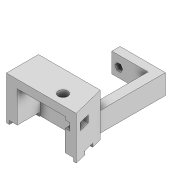
# Autodesk Inventor part: Part2
Saved by Autodesk Inventor 2022 (Build 260153000, 153)
## iProperties
Created: 2021-06-22
Part Number: Part2
Material: Generic
Document SubType Name: Modeling
Designer: Prajwal Patil
Density: 1 g/cm^3
Appearance: Default
Author: Prajwal Patil
Autodesk Inventor part; units mm, degrees
ref_plane "YZ Plane" through (0, 0, 0) normal (1, 0, 0) x (0, 1, 0)
ref_plane "XZ Plane" through (0, 0, 0) normal (0, 1, 0) x (-1, 0, 0)
sketch "Sketch1" plane through (0, 0, 0) normal (0, 0, 1) x (1, 0, 0)
  line L0 (-33.8514, 24.552) -> (33.4586, 24.552)
  line L1 (33.4586, 24.552) -> (33.4586, -22.438)
  line L2 (33.4586, -22.438) -> (-33.8514, -22.438)
  line L3 (-33.8514, -22.438) -> (-33.8514, 24.552)
  line L4 (33.4586, -22.438) -> (33.4586, -16.088)
  line L5 (33.4586, -16.088) -> (23.2986, -16.088)
  line L6 (23.2986, -16.088) -> (23.2986, 5.502)
  line L7 (23.2986, 5.502) -> (33.4586, 5.502)
  point P0 (0, 0)
  dimension "d0" = 67.31
  dimension "d1" = 46.99
  dimension "d10" = 6.35
  dimension "d11" = 10.16
  dimension "d12" = 21.59
  constraints: 16 end point, 4 perpendicular, 2 parallel, 2 point on line, 1 horizontal
  measures "d0" distance of L1.end L2.end
  measures "d1" distance of L0.end L1.end
  measures "d10" distance of L1.end L4.end
  measures "d11" distance of L4.end L5.end
  measures "d12" distance of L5.end L6.end
ref_plane "Work Plane3" through (-33.8514, -22.438, 0) normal (0, 0, 1) x (0, 1, 0)
ref_plane "Work Plane4" through (-33.8514, -22.438, 35.052) normal (0, 0, 1) x (0, 1, 0)
sketch "Sketch3" plane through (-33.8514, -22.438, 35.052) normal (0, 0, 1) x (0, 1, 0)
  line L0 (0, 0) -> (46.99, 0)
  line L1 (46.99, 0) -> (46.99, -76.2)
  line L2 (46.99, -76.2) -> (0, -76.2)
  line L3 (0, -76.2) -> (0, 0)
  point P0 (22.438, -33.8514)
  dimension "d4" = 46.99
  dimension "d5" = 76.2
  constraints: 8 end point, 2 parallel, 1 horizontal, 1 perpendicular
  measures "d4" distance of L1.end L2.end
  measures "d5" distance of L0.end L1.end
loft "Loft1" add profiles "Sketch3", "Sketch1"
sketch "Sketch5" plane through (33.4586, -22.438, 0) normal (0, 0, -1) x (-1, 0, 0)
  line L0 (67.31, 0) -> (67.31, 46.99) projected
  line L1 (-8.89, 0) -> (67.31, 0) projected
  circle A0 centre (42.037, 16.383) radius 3.683
  circle A1 centre (42.037, 16.383) radius 2.159
  point P0 (33.4586, 22.438)
  dimension "d17" = 7.366
  dimension "d20" = 4.318
  constraints: 2 centre point, 1 coincident
  measures "d17" diameter of A0
  measures "d20" diameter of A1
extrude "Extrusion1" add sketch "Sketch1" against normal blind 71.12 contours L1 L5 L6 L7
extrude "Extrusion4" cut sketch "Sketch5" along normal through all both and the other way through all contours A1
extrude "Extrusion5" cut sketch "Sketch5" against normal blind 3.81 contours A0 | A1
sketch "Sketch7" plane through (23.2986, -16.088, 0) normal (-1, 0, 0) x (0, 0, 1)
  point P0 (0, 16.088)
sketch "Sketch8" plane through (23.2986, -16.088, 0) normal (-1, 0, 0) x (0, 0, 1)
  line L0 (0, 0) -> (-71.12, 0) projected
  line L1 (0, 21.59) -> (-71.12, 21.59) projected
  line L2 (-71.12, 0) -> (-62.23, 0)
  line L3 (-62.23, 0) -> (-62.23, 21.59)
  line L4 (-62.23, 21.59) -> (-71.12, 21.59)
  line L5 (-71.12, 21.59) -> (-71.12, 0)
  point P0 (0, 16.088)
  dimension "d27" = 8.89
  constraints: 8 end point, 2 parallel, 1 horizontal, 1 perpendicular, 1 point on line
  measures "d27" distance of L4.end L3.end
extrude "Extrusion6" add sketch "Sketch8" along normal blind 39.37
sketch "Sketch9" plane through (0, 0, -71.12) normal (0, 0, -1) x (-1, 0, 0)
  line L0 (16.0714, 5.502) -> (16.0714, -16.088) projected
  line L1 (-33.4586, -16.088) -> (16.0714, -16.088) projected
  circle A0 centre (8.5784, -6.055) radius 2.54
  point P0 (0, 0)
  dimension "d34" = 5.08
  constraints: 1 centre point, 1 coincident
  measures "d34" diameter of A0
extrude "Extrusion7" cut sketch "Sketch9" against normal blind 39.37
sketch "Sketch10" plane through (-33.8514, -22.438, 35.052) normal (0, -1, 0) x (1, 0, 0)
  line L0 (67.31, -35.052) -> (67.31, -106.172) projected
  line L1 (67.31, -35.052) -> (70.1199, -23.9728)
  line L2 (76.2, 0) -> (67.31, -35.052) projected
  line L3 (70.1199, -23.9728) -> (64.2779, -23.9728)
  line L4 (64.2779, -23.9728) -> (64.2779, -24.9888)
  line L5 (64.2779, -24.9888) -> (11.9539, -24.9888)
  line L6 (11.9539, -24.9888) -> (11.9539, -23.9728)
  line L7 (11.9539, -23.9728) -> (3.1655, -23.9728)
  line L8 (3.1655, -23.9728) -> (3.1655, 0)
  line L9 (0, 0) -> (76.2, 0) projected
  line L10 (76.2, 0) -> (73.0154, -12.5564)
  line L11 (76.2, 0) -> (73.152, 0)
  line L12 (73.152, 0) -> (73.0154, -12.5564)
  line L13 (73.0154, -12.5564) -> (70.1199, -23.9728)
  line L14 (73.152, 0) -> (3.1655, 0)
  line L15 (11.9539, -23.9728) -> (11.9539, 0)
  line L16 (64.2779, -23.9728) -> (64.2779, 0)
  line L17 (11.9539, 0) -> (7.1279, 0)
  circle A0 centre (7.1279, -5.334) radius 1.27
  line L18 (11.9539, -23.9728) -> (7.1279, -23.9728)
  circle A1 centre (7.1279, -16.3528) radius 1.27
  line L19 (73.152, 0) -> (68.326, 0)
  line L20 (64.2779, 0) -> (69.1039, 0)
  circle A2 centre (69.1039, -5.334) radius 1.27
  line L21 (64.2779, -23.9728) -> (69.1039, -23.9728)
  circle A3 centre (69.1039, -16.3528) radius 1.27
  point P0 (33.8514, -35.052)
  point P1 (64.2779, 0)
  point P2 (11.9539, 0)
  dimension "d37" = 11.43
  dimension "d38" = 5.842
  dimension "d39" = 1.016
  dimension "d40" = 52.324
  dimension "d41" = 8.7884
  dimension "d42" = 12.954
  dimension "d43" = 3.048
  dimension "d48" = 4.826
  dimension "d50" = 2.54
  dimension "d52" = 2.54
  dimension "d56" = 4.826
  dimension "d58" = 2.54
  dimension "d59" = 4.826
  dimension "d61" = 2.54
  constraints: 38 end point, 13 point on line, 6 perpendicular, 4 centre point, 2 collinear, 1 horizontal
  measures "d37" distance of L0.start L1.end
  measures "d38" distance of L1.end L3.end
  measures "d39" distance of L3.end L4.end
  measures "d40" distance of L4.end L5.end
  measures "d41" distance of L6.end L7.end
  measures "d42" distance of L2.start L10.end
  measures "d43" distance of L2.start L11.end
  measures "d48" distance of L15.end L17.end
  measures "d50" diameter of A0
  measures "d52" diameter of A1
  measures "d56" distance of L16.end L20.end
  measures "d58" diameter of A2
  measures "d59" distance of L3.end L21.end
  measures "d61" diameter of A3
extrude "Extrusion8" cut sketch "Sketch10" against normal blind 38.1 contours L4 L5 L6 L15 L9 L16
extrude "Extrusion9" cut sketch "Sketch10" against normal blind 3.81 contours L2 L3 L16 L9 L12 | L15 L7 L8 L9 | A0 | A1 | A2 | A3
sketch "Sketch15" plane through (-33.8514, -18.628, 35.052) normal (0, -1, 0) x (1, 0, 0)
  line L0 (11.9539, -24.9888) -> (11.9539, 0) projected
  line L1 (11.9539, -23.9729) -> (11.9539, -16.3529)
  line L2 (11.9539, -16.3529) -> (7.1279, -16.3529)
  circle A0 centre (7.1279, -16.3529) radius 1.27
  line L3 (11.9539, 0) -> (64.2779, 0) projected
  line L4 (11.9539, 0) -> (7.1279, 0)
  line L5 (3.1655, 0) -> (11.9539, 0) projected
  circle A1 centre (7.1279, -5.334) radius 1.27
  point P0 (33.8514, -35.052)
  dimension "d64" = 7.62
  dimension "d65" = 4.826
  dimension "d66" = 2.54
  dimension "d70" = 2.54
  constraints: 6 end point, 3 point on line, 2 centre point, 1 coincident, 1 horizontal
  measures "d64" distance of L1.start L1.end
  measures "d65" distance of L1.end L2.end
  measures "d66" diameter of A0
  measures "d70" diameter of A1
extrude "Extrusion11" cut sketch "Sketch15" against normal blind 10.16 contours A0
sketch "Sketch14" plane through (-33.8514, -18.628, 35.052) normal (0, -1, 0) x (1, 0, 0)
  point P0 (33.8514, -35.052)
extrude "Extrusion12" cut sketch "Sketch15" against normal blind 10.16 contours A1
sketch "Sketch16" plane through (-33.8514, -18.628, 35.052) normal (0, -1, 0) x (1, 0, 0)
  line L0 (11.9539, 0) -> (64.2779, 0) projected
  line L1 (64.2779, 0) -> (69.1039, 0)
  line L2 (0, 0) -> (76.2, 0) projected
  circle A0 centre (69.1039, -5.334) radius 1.27
  line L3 (64.2779, -23.9728) -> (64.2779, -24.9888) projected
  line L4 (64.2779, -23.9728) -> (69.1039, -23.9728)
  line L5 (70.1199, -23.9728) -> (64.2779, -23.9728) projected
  circle A1 centre (69.1039, -16.3528) radius 1.27
  point P0 (33.8514, -35.052)
  dimension "d73" = 4.826
  dimension "d75" = 2.54
  dimension "d76" = 4.826
  dimension "d78" = 2.54
  constraints: 4 end point, 2 centre point, 2 point on line
  measures "d73" distance of L0.end L1.end
  measures "d75" diameter of A0
  measures "d76" distance of L3.start L4.end
  measures "d78" diameter of A1
extrude "Extrusion13" cut sketch "Sketch16" against normal blind 10.16
sketch "Sketch17" plane through (-33.8514, 15.662, 35.052) normal (0, -1, 0) x (1, 0, 0)
  line L0 (64.2779, -23.9728) -> (64.2779, 0) projected
  line L1 (64.2779, 0) -> (50.3079, 0)
  line L2 (11.9539, 0) -> (64.2779, 0) projected
  circle A0 centre (50.3079, -11.43) radius 3.81
  point P0 (33.8514, -35.052)
  dimension "d81" = 13.97
  dimension "d83" = 7.62
  constraints: 2 end point, 1 centre point, 1 point on line
  measures "d81" distance of L0.end L1.end
  measures "d83" diameter of A0
extrude "Extrusion14" cut sketch "Sketch17" against normal through all
sketch "Sketch18" plane through (-33.8514, 24.552, 35.052) normal (0, 1, 0) x (1, 0, 0)
  circle A0 centre (50.3079, 11.43) radius 3.81 projected
  circle A1 centre (50.3079, 11.43) radius 5.207
  point P0 (33.8514, 35.052)
  dimension "d86" = 10.414
  constraints: 1 centre point, 1 coincident
  measures "d86" diameter of A1
extrude "Extrusion15" cut sketch "Sketch18" against normal blind 6.35 contours A0 | A1
sketch "Sketch19" plane through (30.4266, -22.438, 10.0632) normal (-1, 0, 0) x (0, 0, 1)
  line L0 (24.9888, 38.1) -> (0, 38.1) projected
  line L1 (24.9888, 38.1) -> (24.9888, 3.81) projected
  line L2 (24.9888, 34.798) -> (7.7168, 34.798)
  line L3 (7.7168, 34.798) -> (7.7168, 27.178)
  line L4 (7.7168, 27.178) -> (24.9888, 27.178)
  point P0 (-10.0632, 22.438)
  dimension "d89" = 3.302
  dimension "d90" = 17.272
  dimension "d91" = 7.62
  constraints: 6 end point, 2 point on line, 1 horizontal, 1 perpendicular, 1 vertical
  measures "d89" distance of L0.start L2.start
  measures "d90" distance of L2.start L2.end
  measures "d91" distance of L2.end L3.end
extrude "Extrusion16" cut sketch "Sketch19" against normal blind 5.08
sketch "Sketch20" plane through (42.3486, -22.438, 35.052) normal (0.9693105, 0, -0.2458396) x (-0.2458396, 0, -0.9693105)
  line L0 (0, 46.99) -> (36.1618, 46.99) projected
  line L1 (0, 46.99) -> (0, 34.798)
  line L2 (0, 46.99) -> (0, 0) projected
  line L3 (0, 34.798) -> (5.842, 34.798) construction
  line L4 (5.842, 34.798) -> (5.842, 27.178)
  line L5 (5.842, 27.178) -> (17.526, 27.178)
  line L6 (17.526, 27.178) -> (17.526, 34.798)
  line L7 (17.526, 34.798) -> (5.842, 34.798)
  point P0 (44.3872, 22.438)
  dimension "d94" = 12.192
  dimension "d98" = 11.684
  constraints: 12 end point, 1 horizontal, 1 perpendicular, 1 point on line
  measures "d94" distance of L0.start L1.end
  measures "d98" distance of L4.end L5.end
extrude "Extrusion17" cut sketch "Sketch20" against normal blind 11.938
sketch "Sketch21" plane through (35.5066, -22.438, 10.0632) normal (-1, 0, 0) x (0, 0, 1)
  line L0 (7.7168, 27.178) -> (7.7168, 34.798) projected
  line L1 (7.7168, 34.798) -> (8.6432, 34.798) projected
  line L2 (7.7168, 34.798) -> (8.6432, 34.798)
  line L3 (8.6432, 27.178) -> (8.6432, 34.798) projected
  line L4 (8.6432, 34.798) -> (8.6432, 27.178)
  line L5 (24.9888, 27.178) -> (7.7168, 27.178) projected
  line L6 (8.6432, 27.178) -> (7.7168, 27.178)
  line L7 (7.7168, 27.178) -> (7.7168, 34.798)
  point P0 (-10.0632, 22.438)
  constraints: 8 end point, 2 collinear, 2 perpendicular
extrude "Extrusion18" cut sketch "Sketch21" against normal blind 11.938
sketch "Sketch22" plane through (23.2986, -16.088, -62.23) normal (0, 0, 1) x (1, 0, 0)
  circle A0 centre (-31.877, 10.033) radius 2.54 projected
  line L0 (-29.5969, 6.3661) -> (-33.9126, 6.2249)
  line L1 (-33.9126, 6.2249) -> (-36.1927, 9.8919)
  line L2 (-36.1927, 9.8919) -> (-34.1571, 13.6999)
  line L3 (-34.1571, 13.6999) -> (-29.8414, 13.8411)
  line L4 (-29.8414, 13.8411) -> (-27.5613, 10.1741)
  line L5 (-27.5613, 10.1741) -> (-29.5969, 6.3661)
  point P0 (-23.2986, 16.088)
  constraints: 12 end point, 1 coincident, 13 other
extrude "Extrusion20" cut sketch "Sketch22" against normal blind 5.08 contours A0 | L0 L1 L2 L3 L4 L5
body "Solid1"
